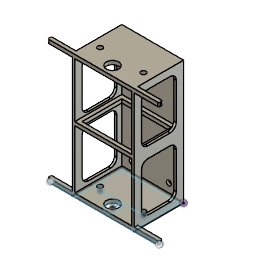
ensamble2 (Autodesk Fusion 360 archive; units mm, degrees)
design "Soporte_Motor_Step28BYJ"
Autodesk Fusion 360 part; units mm, degrees
sketch "Sketch1" plane through (0, 0, 0) normal (0, 1, 0) x (1, 0, 0)
  line L0 (0, 0) -> (-50, 0)
  line L1 (-50, 0) -> (-50, -25)
  line L2 (-50, -25) -> (-50, -40)
  line L3 (-25, -25) -> (-42.5, -25)
  line L4 (-25, -25) -> (-7.5, -25)
  circle A0 centre (-42.5, -25) radius 2
  circle A1 centre (-7.5, -25) radius 2
  line L5 (-25, -25) -> (-25, -32.5)
  circle A2 centre (-25, -32.5) radius 5
  line L6 (-50, -40) -> (0, -40)
  line L7 (0, -40) -> (0, 0)
  line L8 (0, -40) -> (19, -40)
  line L9 (20, -39) -> (20, -38)
  line L10 (19, -37) -> (0, -37)
  line L11 (-50, -40) -> (-69, -40)
  line L12 (-70, -39) -> (-70, -38)
  line L13 (-69, -37) -> (-50, -37)
  arc A3 (20, -38) -> (19, -37) centre (19, -38) ccw
  arc A4 (19, -40) -> (20, -39) centre (19, -39) ccw
  arc A5 (-70, -39) -> (-69, -40) centre (-69, -39) ccw
  arc A6 (-69, -37) -> (-70, -38) centre (-69, -38) ccw
  line L14 (-50, -2) -> (0, -2)
  line L15 (-48, 0) -> (-48, -40)
  line L16 (-2, 0) -> (-2, -40)
  dimension "d1" = 50
  dimension "d2" = 15
  dimension "d3" = 17.5
  dimension "d5" = 17.5
  dimension "d7" = 4
  dimension "d8" = 4
  dimension "d9" = 7.5
  dimension "d10" = 10
  dimension "d11" = 1
  constraint coincident L0.start L7.end
  constraint horizontal L0
  constraint perpendicular L0 L1
  constraint parallel L1 L2
  constraint perpendicular L1 L3
  constraint parallel L3 L4
  constraint coincident L3.end A0.centre
  constraint coincident L4.end A1.centre
  constraint perpendicular L4 L5
  constraint coincident L5.end A2.centre
  constraint perpendicular L2 L6
  constraint perpendicular L0 L7
  constraint perpendicular L7 L8
  constraint perpendicular L8 L9
  constraint coincident L7 L10.end
  constraint perpendicular L7 L10
  constraint perpendicular L2 L11
  constraint perpendicular L11 L12
  constraint coincident L2 L13.end
  constraint perpendicular L2 L13
  constraint tangent L10 A3
  constraint tangent L9 A3
  constraint tangent L8 A4
  constraint tangent L9 A4
  constraint equal A3 A4
  constraint tangent L11 A5
  constraint tangent L12 A5
  constraint equal A3 A5
  constraint tangent L12 A6
  constraint tangent L13 A6
  constraint equal A3 A6
  constraint coincident L1 L14.start
  constraint coincident L7 L14.end
  constraint perpendicular L7 L14
  constraint coincident L0 L15.start
  constraint coincident L6 L15.end
  constraint perpendicular L6 L15
  constraint coincident L0 L16.start
  constraint coincident L6 L16.end
  constraint perpendicular L6 L16
  measures "d1" distance of L0.start L0.end
  measures "d2" distance of L1.end L2.end
  measures "d3" distance of L3.start L3.end
  measures "d5" distance of L3.start L4.end
  measures "d7" diameter of A0
  measures "d8" diameter of A1
  measures "d9" distance of L3.start L5.end
  measures "d10" diameter of A2
  measures "d11" radius of A3
extrude "Extrude1" add sketch "Sketch1" along normal blind 3
extrude "Extrude2" add sketch "Sketch1" along normal blind 95 from surface at 3 contours L0 L7 L14 L16 | L0 L14 L15 L16 | L6 L7 L14 L16 | L0 L1 L14 L15 | L1 L2 L6 L14 L15
extrude "Extrude3" add sketch "Sketch1" along normal blind 3 from surface at 97
sketch "Sketch2" plane through (0, 100, 0) normal (0, 1, 0) x (-1, 0, 0)
  circle A0 centre (7.5, 25) radius 2
  circle A1 centre (42.5, 25) radius 2
  circle A2 centre (25, 32.5) radius 5
  line L0 (69, 40) -> (-19, 40)
  arc A3 (-19, 40) -> (-20, 39) centre (-19, 39) ccw
  line L1 (-20, 39) -> (-20, 38)
  arc A4 (-20, 38) -> (-19, 37) centre (-19, 38) ccw
  line L2 (-19, 37) -> (0, 37)
  line L3 (0, 37) -> (0, 0)
  line L4 (0, 0) -> (50, 0)
  line L5 (50, 0) -> (50, 37)
  line L6 (50, 37) -> (69, 37)
  arc A5 (69, 37) -> (70, 38) centre (69, 38) ccw
  line L7 (70, 38) -> (70, 39)
  arc A6 (70, 39) -> (69, 40) centre (69, 39) ccw
  line L8 (47, 0) -> (3, 0)
  line L9 (50, 40) -> (50, 0)
  line L10 (0, 0) -> (0, 40)
  line L11 (50, 40) -> (0, 40)
  line L12 (45, 0) -> (45, 5)
  line L13 (45, 5) -> (5, 5)
  line L14 (5, 5) -> (5, 37)
  line L15 (5, 37) -> (45, 37)
  line L16 (45, 37) -> (45, 5)
  constraint horizontal L8
  constraint coincident L4 L8.start
  constraint coincident L0 L9.start
  constraint coincident L4.end L5.start
  constraint coincident L3.end L4.start
  constraint coincident L0 L10.end
  constraint perpendicular L0 L10
  constraint coincident L8 L12.start
  constraint perpendicular L8 L12
  constraint perpendicular L10 L13
  constraint perpendicular L13 L14
  constraint perpendicular L12 L15
  constraint perpendicular L13 L16
extrude "Extrude4" add sketch "Sketch2" against normal blind 3 from surface at -47 contours A2 L15 | L0 L3 L4 L5 L8 L9 L10 L11 picked at (24.8927, 37.1632)
sketch "Sketch3" plane through (0, 0, 0) normal (1, 0, 0) x (0, 0, -1)
  line L0 (-3, 97) -> (-3, 3)
  line L1 (-3, 3) -> (-37, 3)
  line L2 (-37, 3) -> (-37, 97)
  line L3 (-3, 50) -> (-3, 51.5)
  line L4 (-3, 50) -> (-3, 48.5)
  line L5 (-3, 51.5) -> (-37, 51.5)
  line L6 (-3, 48.5) -> (-37, 48.5)
  line L7 (-3, 97) -> (-37, 97)
  line L8 (-6, 89) -> (-6, 59.5)
  line L9 (-11, 94) -> (-29, 94)
  line L10 (-34, 89) -> (-34, 59.5)
  line L11 (-29, 54.5) -> (-11, 54.5)
  line L12 (-40, 50) -> (-2, 50)
  line L13 (-6, 11) -> (-6, 40.5)
  line L14 (-11, 6) -> (-29, 6)
  line L15 (-34, 11) -> (-34, 40.5)
  line L16 (-29, 45.5) -> (-11, 45.5)
  arc A0 (-6, 89) -> (-11, 94) centre (-11, 89) ccw
  arc A1 (-29, 94) -> (-34, 89) centre (-29, 89) ccw
  arc A2 (-34, 59.5) -> (-29, 54.5) centre (-29, 59.5) ccw
  arc A3 (-11, 54.5) -> (-6, 59.5) centre (-11, 59.5) ccw
  arc A4 (-6, 40.5) -> (-11, 45.5) centre (-11, 40.5) ccw
  arc A5 (-29, 45.5) -> (-34, 40.5) centre (-29, 40.5) ccw
  arc A6 (-11, 6) -> (-6, 11) centre (-11, 11) ccw
  arc A7 (-34, 11) -> (-29, 6) centre (-29, 11) ccw
  point P0 (-6, 94)
  point P1 (-6, 54.5)
  dimension "d23" = 1.5
  dimension "d24" = 1.5
  dimension "d25" = 39.5
  dimension "d26" = 5
  dimension "d27" = 5
  dimension "d28" = 5
  dimension "d29" = 5
  dimension "d30" = 5
  dimension "d31" = 5
  dimension "d32" = 5
  constraint vertical L0
  constraint perpendicular L0 L1
  constraint perpendicular L1 L2
  constraint midpoint L0 L3.start
  constraint parallel L0 L3
  constraint parallel L0 L4
  constraint coincident L2 L5.end
  constraint perpendicular L2 L5
  constraint coincident L2 L6.end
  constraint perpendicular L2 L6
  constraint perpendicular L0 L7
  constraint perpendicular L5 L8
  constraint perpendicular L8 L9
  constraint perpendicular L9 L10
  constraint perpendicular L8 L11
  constraint coincident P0 L8
  constraint coincident P0 L9
  constraint tangent L8 A0
  constraint tangent L9 A0
  constraint tangent L9 A1
  constraint tangent L10 A1
  constraint tangent L10 A2
  constraint tangent L11 A2
  constraint equal A1 A2
  constraint coincident P1 L8
  constraint coincident P1 L11
  constraint tangent L8 A3
  constraint tangent L11 A3
  constraint tangent L13 A4
  constraint tangent L16 A4
  constraint tangent L16 A5
  constraint tangent L15 A5
  constraint tangent L13 A6
  constraint tangent L14 A6
  constraint tangent L14 A7
  constraint tangent L15 A7
  measures "d23" distance of L3.start L3.end
  measures "d24" distance of L3.start L4.end
  measures "d25" distance of P0 P1
  measures "d26" radius of A0
  measures "d27" radius of A1
  measures "d28" radius of A3
  measures "d29" radius of A4
  measures "d30" radius of A5
  measures "d31" radius of A6
  measures "d32" radius of A7
extrude "Extrude5" cut sketch "Sketch3" against normal blind 50 contours L8 L9 L10 L11 A0 A1 A2 A3 | L13 L14 L15 L16 A4 A5 A6 A7
sketch "Sketch4" plane through (0, 0, 0) normal (0, 0, 1) x (1, 0, 0)
  circle A0 centre (-10, 10) radius 2
  circle A1 centre (-40, 10) radius 2
  line L0 (-2, 50) -> (-48, 50)
  circle A2 centre (-10, 90) radius 2
  circle A3 centre (-40, 90) radius 2
  dimension "d36" = 4
  dimension "d38" = 4
  constraint symmetric A0 L0 A2
  constraint symmetric A1 L0 A3
  measures "d36" diameter of A0
  measures "d38" diameter of A1
extrude "Extrude6" cut sketch "Sketch4" along normal blind 3

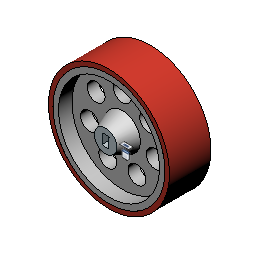
design "Ruedas"
Autodesk Fusion 360 part; units mm, degrees
sketch "Sketch1" plane through (0, 0, 0) normal (0, 1, 0) x (1, 0, 0)
  circle A0 centre (0, 0) radius 25
  dimension "d1" = 50
  constraint coincident A0.centre origin
  measures "d1" diameter of A0
extrude "Extrude1" add sketch "Sketch1" along normal blind 20 makes body 1
sketch "Sketch2" plane through (0, 20, 0) normal (0, 1, 0) x (-1, 0, 0)
  circle A0 centre (0, 0) radius 25
  line L0 (-1.5, 2.0622) -> (-1.5, -2.0622)
  line L1 (1.5, 2.0622) -> (1.5, -2.0622)
  arc A1 (-1.5, -2.0622) -> (1.5, -2.0622) centre (0, 0) ccw
  arc A2 (1.5, 2.0622) -> (-1.5, 2.0622) centre (0, 0) ccw
  dimension "d4" = 5.1
  constraint coincident A0.centre A1.centre
  constraint coincident L1.start A1
  constraint concentric A1 A2
  measures "d4" diameter of A1
extrude "Extrude2" cut sketch "Sketch2" against normal blind 50 contours L0 L1 A1 A2 bodies 1
sketch "Sketch3" plane through (0, 20, 0) normal (0, 1, 0) x (-1, 0, 0)
  line L0 (-1.5, -2.0622) -> (-1.5, 2.0622)
  arc A0 (1.5, 2.0622) -> (-1.5, 2.0622) centre (0, 0) ccw
  line L1 (1.5, 2.0622) -> (1.5, -2.0622)
  arc A1 (-1.5, -2.0622) -> (1.5, -2.0622) centre (0, 0) ccw
  circle A2 centre (0, 0) radius 25
  circle A3 centre (0, 0) radius 5
  circle A4 centre (0, 0) radius 22.5
  dimension "d9" = 45
  constraint coincident A0.centre A1.centre
  measures "d9" diameter of A4
extrude "Extrude3" cut sketch "Sketch3" against normal blind 7.5 contours A4 bodies 1
sketch "Sketch4" plane through (0, 0, 0) normal (0, 1, 0) x (1, 0, 0)
  circle A0 centre (0, 0) radius 5
  circle A1 centre (0, 0) radius 22.5
extrude "Extrude4" cut sketch "Sketch4" along normal blind 7.5 bodies 1
sketch "Sketch5" plane through (0, 12.5, 0) normal (0, 1, 0) x (-1, 0, 0)
  circle A0 centre (0, 0) radius 5
  circle A1 centre (0, 0) radius 22.5
  circle A2 centre (0, 15) radius 4
  circle A3 centre (-11.7275, 9.3523) radius 4
  circle A4 centre (-14.6239, -3.3378) radius 4
  circle A5 centre (-6.5083, -13.5145) radius 4
  circle A6 centre (6.5083, -13.5145) radius 4
  circle A7 centre (14.6239, -3.3378) radius 4
  circle A8 centre (11.7275, 9.3523) radius 4
  dimension "d15" = 360
  dimension "d16" = 8
  measures "d16" diameter of A2
extrude "Extrude5" cut sketch "Sketch5" against normal blind 9 contours A2 | A3 | A4 | A5 | A6 | A7 | A8 bodies 1
extrude "Extrude6" cut 1 faces at (2.6667, 20, 0) along direction (0, -1, 0) blind 7.5 on bodies 1 bodies 1
extrude "Extrude7" cut 1 faces at (23.9898, 0, 2.3598) along direction (0, 1, 0) blind 1.5 on bodies 1 bodies 1
sketch "Sketch6" plane through (0, 12.5, 0) normal (0, 1, 0) x (-1, 0, 0)
  line L0 (-1.5, -2.0622) -> (-1.5, 2.0622)
  arc A0 (1.5, 2.0622) -> (-1.5, 2.0622) centre (0, 0) ccw
  line L1 (1.5, 2.0622) -> (1.5, -2.0622)
  arc A1 (-1.5, -2.0622) -> (1.5, -2.0622) centre (0, 0) ccw
  circle A2 centre (6.5083, -13.5145) radius 4
  circle A3 centre (0, 15) radius 4
  circle A4 centre (-6.5083, -13.5145) radius 4
  circle A5 centre (14.6239, -3.3378) radius 4
  circle A6 centre (-11.7275, 9.3523) radius 4
  circle A7 centre (-14.6239, -3.3378) radius 4
  circle A8 centre (11.7275, 9.3523) radius 4
  circle A9 centre (0, 0) radius 22.5
  arc A10 (1.5, 2.0622) -> (-1.5, 2.0622) centre (0, 0) ccw
  line L2 (-1.5, 2.0622) -> (-1.5, -2.0622)
  arc A11 (-1.5, -2.0622) -> (1.5, -2.0622) centre (0, 0) ccw
  line L3 (1.5, 2.0622) -> (1.5, -2.0622)
extrude "Extrude8" add sketch "Sketch6" against normal blind 7.5 contours L0 A0 L1 A1 A10 L2 A11 L3 bodies 1
chamfer "Chamfer1" distance 7.5 distance2 3 1 edges at (-4.6616, 7.5, -1.8081) measured on face at (4.9752, 5, 0.4978) on bodies 1
sketch "Sketch7" plane through (0, 0, 0) normal (0, -1, 0) x (1, 0, 0)
  circle A0 centre (0, 0) radius 5
  line L0 (1.5, 2.0622) -> (1.5, -2.0622)
  arc A1 (-1.5, -2.0622) -> (1.5, -2.0622) centre (0, 0) ccw
  line L1 (-1.5, -2.0622) -> (-1.5, 2.0622)
  arc A2 (1.5, 2.0622) -> (-1.5, 2.0622) centre (0, 0) ccw
sketch "Sketch8" plane through (0, 20, 0) normal (0, 1, 0) x (-1, 0, 0)
  circle A0 centre (0, 0) radius 25
  circle A1 centre (0, 0) radius 22.5
  circle A2 centre (0, 0) radius 27
  circle A3 centre (0, 0) radius 25
  dimension "d27" = 54
  dimension "d28" = 50
  constraint coincident A0.centre A1.centre
  measures "d27" diameter of A2
  measures "d28" diameter of A3
extrude "Extrude9" add sketch "Sketch8" against normal blind 18.5 separate body contours A2 makes body 2
